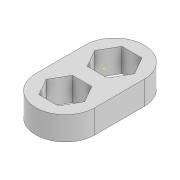
# Autodesk Inventor part: Sujeción venturi a ventosa
Saved by Autodesk Inventor 2022 (Build 260153000, 153)
## iProperties
Created: 2022-10-26
Part Number: Sujeción venturi a ventosa
Material: Generic
Document SubType Name: Modeling
Designer: ADMIN
Density: 1 g/cm^3
Appearance: Default
Author: ADMIN
## iProperties of the stored document Sujeción venturi a ventosa_3DPrint.ipt
Created: 2022-10-26
Part Number: Sujeción venturi a ventosa_3DPrint
Material: Generic
Document SubType Name: Modeling
Designer: ADMIN
Density: 1 g/cm^3
Appearance: Default
Author: ADMIN
Autodesk Inventor part; units mm, degrees
ref_plane "YZ Plane" through (0, 0, 0) normal (1, 0, 0) x (0, 1, 0)
ref_plane "XZ Plane" through (0, 0, 0) normal (0, 1, 0) x (-1, 0, 0)
ref_plane "XY Plane" through (0, 0, 0) normal (0, 0, 1) x (1, 0, 0)
sketch "Sketch1" plane through (0, 0, 0) normal (0, 1, 0) x (-1, 0, 0)
  line L0 (-9.6523, 19.392) -> (-4.7448, 27.892)
  line L1 (-4.7448, 27.892) -> (5.0701, 27.892)
  line L2 (5.0701, 27.892) -> (9.9776, 19.392)
  line L3 (9.9776, 19.392) -> (5.0701, 10.892)
  line L4 (5.0701, 10.892) -> (-4.7448, 10.892)
  line L5 (-4.7448, 10.892) -> (-9.6523, 19.392)
  line L6 (-4.918, -14.408) -> (-9.9987, -5.608)
  line L7 (-9.9987, -5.608) -> (-4.918, 3.192)
  line L8 (-4.918, 3.192) -> (5.2433, 3.192)
  line L9 (5.2433, 3.192) -> (10.324, -5.608)
  line L10 (10.324, -5.608) -> (5.2433, -14.408)
  line L11 (5.2433, -14.408) -> (-4.918, -14.408)
  line L12 (-8.4421, 41.1326) -> (9.2977, 41.1326)
  line L13 (15.1626, 19.392) -> (15.1626, -5.608)
  line L14 (-14.8374, 19.392) -> (-14.8374, -5.608)
  arc A0 (-14.8374, -5.608) -> (15.1626, -5.608) centre (0.1626, -5.608) ccw
  arc A1 (15.1626, 19.392) -> (-14.8374, 19.392) centre (0.1626, 19.392) ccw
  point P0 (0, 0)
  dimension "d0" = 8.5
  dimension "d1" = 8.8
  dimension "d2" = 25
  dimension "d5" = 15
  constraints: 30 end point, 4 point on circle, 3 parallel, 3 tangent, 2 centre point, 2 coincident, 1 horizontal, 1 vertical, 26 other
  measures "d0" distance from line of L4 point (0.163, 19.392)
  measures "d1" distance from line of L11 point (0.163, -5.608)
  measures "d2" distance of point (0.163, -5.608) point (0.163, 19.392)
  measures "d5" radius of A1
extrude "Extrusion1" add sketch "Sketch1" along normal blind 12
sketch "Sketch2" plane through (0, 12, 0) normal (0, 1, 0) x (1, 0, 0)
  point P0 (0, 0)
body "Solid1"
